Autodesk Fusion 360 part; units mm, degrees
(part 3 of 5)
  arc A39 (-57.6679, 11.8099) -> (-56.8988, 12.9306) centre (-57.8882, 12.7853) ccw
  arc A40 (-57.6679, 11.8099) -> (-58.5945, 11.5616) centre (-55, 0) ccw
  arc A41 (-59.8209, 12.1477) -> (-58.5945, 11.5616) centre (-58.8914, 12.5165) ccw
  line L20 (-59.8209, 12.1477) -> (-60.1994, 13.1014)
  spline S20 degree 5 poles (-60.1994, 13.1014) (-60.2031, 13.1108) (-60.2109, 13.1295) (-60.2234, 13.1571) (-60.2418, 13.1932) (-60.267, 13.2372) (-60.2939, 13.2804) (-60.3217, 13.3231) (-60.3501, 13.3657) (-60.3789, 13.408) (-60.4081, 13.4502) (-60.4379, 13.4921) (-60.4683, 13.5336) (-60.4995, 13.5747) (-60.5315, 13.6155) (-60.5642, 13.6558) (-60.5976, 13.6958) (-60.6314, 13.7355) (-60.6658, 13.775) (-60.7005, 13.8143) (-60.7357, 13.8532) (-60.7713, 13.8919) (-60.8074, 13.9304) (-60.844, 13.9685) (-60.8811, 14.0064) (-60.9187, 14.044) (-60.9566, 14.0813) (-60.995, 14.1184) (-61.0338, 14.1552) (-61.073, 14.1917) (-61.1126, 14.228) (-61.1525, 14.2641) (-61.1929, 14.2999) (-61.2336, 14.3354) (-61.2747, 14.3707) (-61.3161, 14.4057) (-61.358, 14.4405) (-61.4002, 14.4751) (-61.4427, 14.5093) (-61.4856, 14.5434) (-61.5288, 14.5772) (-61.5723, 14.6107) (-61.6162, 14.644) (-61.6604, 14.6771) (-61.7049, 14.7099) (-61.7498, 14.7424) (-61.7949, 14.7747) (-61.8404, 14.8068) (-61.8862, 14.8386) (-61.9323, 14.8702) (-61.9787, 14.9015) (-62.0253, 14.9326) (-62.0723, 14.9634) (-62.1196, 14.994) (-62.1672, 15.0244) (-62.215, 15.0545) (-62.2631, 15.0843) (-62.3115, 15.114) (-62.3602, 15.1433) (-62.4092, 15.1724) (-62.4584, 15.2013) (-62.5079, 15.2299) (-62.5577, 15.2583) (-62.6077, 15.2865) (-62.658, 15.3143) (-62.7085, 15.342) (-62.7594, 15.3694) (-62.8104, 15.3965) (-62.8617, 15.4234) (-62.9133, 15.4501) (-62.9651, 15.4765) (-63.0067, 15.4974) (-63.038, 15.513) (-63.059, 15.5233) (-63.0695, 15.5285) knots 0 0 0 0 0 0 0.01428571 0.02857143 0.04285714 0.05714286 0.07142857 0.08571429 0.1 0.11428571 0.12857143 0.14285714 0.15714286 0.17142857 0.18571429 0.2 0.21428571 0.22857143 0.24285714 0.25714286 0.27142857 0.28571429 0.3 0.31428571 0.32857143 0.34285714 0.35714286 0.37142857 0.38571429 0.4 0.41428571 0.42857143 0.44285714 0.45714286 0.47142857 0.48571429 0.5 0.51428571 0.52857143 0.54285714 0.55714286 0.57142857 0.58571429 0.6 0.61428571 0.62857143 0.64285714 0.65714286 0.67142857 0.68571429 0.7 0.71428571 0.72857143 0.74285714 0.75714286 0.77142857 0.78571429 0.8 0.81428571 0.82857143 0.84285714 0.85714286 0.87142857 0.88571429 0.9 0.91428571 0.92857143 0.94285714 0.95714286 0.97142857 0.98571429 1 1 1 1 1 1
  arc A42 (-63.0695, 15.5285) -> (-64.4133, 14.7526) centre (-55, 0) ccw
  spline S21 degree 5 poles (-64.4133, 14.7526) (-64.4141, 14.741) (-64.4156, 14.7176) (-64.4178, 14.6827) (-64.4205, 14.6362) (-64.4235, 14.5781) (-64.4262, 14.5202) (-64.4286, 14.4623) (-64.4306, 14.4045) (-64.4323, 14.3468) (-64.4336, 14.2892) (-64.4346, 14.2317) (-64.4353, 14.1743) (-64.4356, 14.117) (-64.4355, 14.0598) (-64.4351, 14.0028) (-64.4344, 13.9458) (-64.4333, 13.889) (-64.4319, 13.8322) (-64.4301, 13.7756) (-64.4279, 13.7191) (-64.4254, 13.6628) (-64.4226, 13.6065) (-64.4193, 13.5504) (-64.4158, 13.4945) (-64.4118, 13.4386) (-64.4075, 13.3829) (-64.4029, 13.3274) (-64.3978, 13.2719) (-64.3924, 13.2167) (-64.3867, 13.1616) (-64.3805, 13.1066) (-64.374, 13.0518) (-64.3671, 12.9971) (-64.3598, 12.9427) (-64.3522, 12.8883) (-64.3441, 12.8342) (-64.3357, 12.7802) (-64.3269, 12.7264) (-64.3177, 12.6728) (-64.3081, 12.6194) (-64.298, 12.5662) (-64.2876, 12.5131) (-64.2768, 12.4603) (-64.2655, 12.4077) (-64.2539, 12.3552) (-64.2418, 12.303) (-64.2293, 12.251) (-64.2164, 12.1993) (-64.2031, 12.1477) (-64.1893, 12.0964) (-64.1751, 12.0454) (-64.1603, 11.9946) (-64.1451, 11.9441) (-64.1294, 11.8939) (-64.1132, 11.8439) (-64.0966, 11.7942) (-64.0796, 11.7447) (-64.0621, 11.6955) (-64.0442, 11.6467) (-64.0256, 11.5981) (-64.0063, 11.5501) (-63.9863, 11.5025) (-63.9655, 11.4554) (-63.9441, 11.4087) (-63.9222, 11.3623) (-63.8999, 11.3162) (-63.8773, 11.2703) (-63.8542, 11.2248) (-63.8302, 11.1799) (-63.8047, 11.1361) (-63.7827, 11.1022) (-63.765, 11.0775) (-63.7527, 11.0614) (-63.7464, 11.0535) knots -1 -1 -1 -1 -1 -1 -0.98571429 -0.97142857 -0.95714286 -0.94285714 -0.92857143 -0.91428571 -0.9 -0.88571429 -0.87142857 -0.85714286 -0.84285714 -0.82857143 -0.81428571 -0.8 -0.78571429 -0.77142857 -0.75714286 -0.74285714 -0.72857143 -0.71428571 -0.7 -0.68571429 -0.67142857 -0.65714286 -0.64285714 -0.62857143 -0.61428571 -0.6 -0.58571429 -0.57142857 -0.55714286 -0.54285714 -0.52857143 -0.51428571 -0.5 -0.48571429 -0.47142857 -0.45714286 -0.44285714 -0.42857143 -0.41428571 -0.4 -0.38571429 -0.37142857 -0.35714286 -0.34285714 -0.32857143 -0.31428571 -0.3 -0.28571429 -0.27142857 -0.25714286 -0.24285714 -0.22857143 -0.21428571 -0.2 -0.18571429 -0.17142857 -0.15714286 -0.14285714 -0.12857143 -0.11428571 -0.1 -0.08571429 -0.07142857 -0.05714286 -0.04285714 -0.02857143 -0.01428571 0 0 0 0 0 0
  line L21 (-63.7464, 11.0535) -> (-63.1097, 10.2488)
  arc A43 (-63.2154, 8.8938) -> (-63.1097, 10.2488) centre (-63.8939, 9.6283) ccw
  arc A44 (-63.2154, 8.8938) -> (-63.8938, 8.2154) centre (-55, 0) ccw
  arc A45 (-65.2488, 8.1097) -> (-63.8938, 8.2154) centre (-64.6283, 8.8939) ccw
  line L22 (-65.2488, 8.1097) -> (-66.0535, 8.7464)
  spline S22 degree 5 poles (-66.0535, 8.7464) (-66.0614, 8.7527) (-66.0775, 8.765) (-66.1022, 8.7827) (-66.1361, 8.8047) (-66.1799, 8.8302) (-66.2248, 8.8542) (-66.2703, 8.8773) (-66.3162, 8.8999) (-66.3623, 8.9222) (-66.4087, 8.9441) (-66.4554, 8.9655) (-66.5025, 8.9863) (-66.5501, 9.0063) (-66.5981, 9.0256) (-66.6467, 9.0442) (-66.6955, 9.0621) (-66.7447, 9.0796) (-66.7942, 9.0966) (-66.8439, 9.1132) (-66.8939, 9.1294) (-66.9441, 9.1451) (-66.9946, 9.1603) (-67.0454, 9.1751) (-67.0964, 9.1893) (-67.1477, 9.2031) (-67.1993, 9.2164) (-67.251, 9.2293) (-67.303, 9.2418) (-67.3552, 9.2539) (-67.4077, 9.2655) (-67.4603, 9.2768) (-67.5131, 9.2876) (-67.5662, 9.298) (-67.6194, 9.3081) (-67.6728, 9.3177) (-67.7264, 9.3269) (-67.7802, 9.3357) (-67.8342, 9.3441) (-67.8883, 9.3522) (-67.9427, 9.3598) (-67.9971, 9.3671) (-68.0518, 9.374) (-68.1066, 9.3805) (-68.1616, 9.3867) (-68.2167, 9.3924) (-68.2719, 9.3978) (-68.3274, 9.4029) (-68.3829, 9.4075) (-68.4386, 9.4118) (-68.4945, 9.4158) (-68.5504, 9.4193) (-68.6065, 9.4226) (-68.6628, 9.4254) (-68.7191, 9.4279) (-68.7756, 9.4301) (-68.8322, 9.4319) (-68.889, 9.4333) (-68.9458, 9.4344) (-69.0028, 9.4351) (-69.0598, 9.4355) (-69.117, 9.4356) (-69.1743, 9.4353) (-69.2317, 9.4346) (-69.2892, 9.4336) (-69.3468, 9.4323) (-69.4045, 9.4306) (-69.4623, 9.4286) (-69.5202, 9.4262) (-69.5781, 9.4235) (-69.6362, 9.4205) (-69.6827, 9.4178) (-69.7176, 9.4156) (-69.741, 9.4141) (-69.7526, 9.4133) knots 0 0 0 0 0 0 0.01428571 0.02857143 0.04285714 0.05714286 0.07142857 0.08571429 0.1 0.11428571 0.12857143 0.14285714 0.15714286 0.17142857 0.18571429 0.2 0.21428571 0.22857143 0.24285714 0.25714286 0.27142857 0.28571429 0.3 0.31428571 0.32857143 0.34285714 0.35714286 0.37142857 0.38571429 0.4 0.41428571 0.42857143 0.44285714 0.45714286 0.47142857 0.48571429 0.5 0.51428571 0.52857143 0.54285714 0.55714286 0.57142857 0.58571429 0.6 0.61428571 0.62857143 0.64285714 0.65714286 0.67142857 0.68571429 0.7 0.71428571 0.72857143 0.74285714 0.75714286 0.77142857 0.78571429 0.8 0.81428571 0.82857143 0.84285714 0.85714286 0.87142857 0.88571429 0.9 0.91428571 0.92857143 0.94285714 0.95714286 0.97142857 0.98571429 1 1 1 1 1 1
  arc A46 (-69.7526, 9.4133) -> (-70.5285, 8.0695) centre (-55, 0) ccw
  spline S23 degree 5 poles (-70.5285, 8.0695) (-70.5233, 8.059) (-70.513, 8.038) (-70.4974, 8.0067) (-70.4765, 7.9651) (-70.4501, 7.9133) (-70.4234, 7.8617) (-70.3965, 7.8104) (-70.3694, 7.7594) (-70.342, 7.7085) (-70.3143, 7.658) (-70.2865, 7.6077) (-70.2583, 7.5577) (-70.2299, 7.5079) (-70.2013, 7.4584) (-70.1724, 7.4092) (-70.1433, 7.3602) (-70.114, 7.3115) (-70.0843, 7.2631) (-70.0545, 7.215) (-70.0244, 7.1672) (-69.994, 7.1196) (-69.9634, 7.0723) (-69.9326, 7.0253) (-69.9015, 6.9787) (-69.8702, 6.9323) (-69.8386, 6.8862) (-69.8068, 6.8404) (-69.7747, 6.7949) (-69.7424, 6.7498) (-69.7099, 6.7049) (-69.6771, 6.6604) (-69.644, 6.6162) (-69.6107, 6.5723) (-69.5772, 6.5288) (-69.5434, 6.4856) (-69.5093, 6.4427) (-69.4751, 6.4002) (-69.4405, 6.358) (-69.4057, 6.3161) (-69.3707, 6.2747) (-69.3354, 6.2336) (-69.2999, 6.1929) (-69.2641, 6.1525) (-69.228, 6.1126) (-69.1917, 6.073) (-69.1552, 6.0338) (-69.1184, 5.995) (-69.0813, 5.9566) (-69.044, 5.9187) (-69.0064, 5.8811) (-68.9685, 5.844) (-68.9304, 5.8074) (-68.8919, 5.7713) (-68.8532, 5.7357) (-68.8143, 5.7005) (-68.775, 5.6658) (-68.7355, 5.6314) (-68.6958, 5.5976) (-68.6558, 5.5642) (-68.6155, 5.5315) (-68.5747, 5.4995) (-68.5336, 5.4683) (-68.4921, 5.4379) (-68.4502, 5.4081) (-68.408, 5.3789) (-68.3657, 5.3501) (-68.3231, 5.3217) (-68.2804, 5.2939) (-68.2372, 5.267) (-68.1932, 5.2418) (-68.1571, 5.2234) (-68.1295, 5.2109) (-68.1108, 5.2031) (-68.1014, 5.1994) knots -1 -1 -1 -1 -1 -1 -0.98571429 -0.97142857 -0.95714286 -0.94285714 -0.92857143 -0.91428571 -0.9 -0.88571429 -0.87142857 -0.85714286 -0.84285714 -0.82857143 -0.81428571 -0.8 -0.78571429 -0.77142857 -0.75714286 -0.74285714 -0.72857143 -0.71428571 -0.7 -0.68571429 -0.67142857 -0.65714286 -0.64285714 -0.62857143 -0.61428571 -0.6 -0.58571429 -0.57142857 -0.55714286 -0.54285714 -0.52857143 -0.51428571 -0.5 -0.48571429 -0.47142857 -0.45714286 -0.44285714 -0.42857143 -0.41428571 -0.4 -0.38571429 -0.37142857 -0.35714286 -0.34285714 -0.32857143 -0.31428571 -0.3 -0.28571429 -0.27142857 -0.25714286 -0.24285714 -0.22857143 -0.21428571 -0.2 -0.18571429 -0.17142857 -0.15714286 -0.14285714 -0.12857143 -0.11428571 -0.1 -0.08571429 -0.07142857 -0.05714286 -0.04285714 -0.02857143 -0.01428571 0 0 0 0 0 0
  line L23 (-68.1014, 5.1994) -> (-67.1477, 4.8209)
  arc A47 (-66.5616, 3.5945) -> (-67.1477, 4.8209) centre (-67.5165, 3.8914) ccw
  circle A48 centre (-55, 0) radius 2.6
  line L24 (-50.5903, -1.85) -> (-59.4097, -1.85)
  line L25 (-59.4097, -1.85) -> (-59.4097, 1.85)
  line L26 (-59.4097, 1.85) -> (-50.5903, 1.85)
  line L27 (-50.5903, 1.85) -> (-50.5903, -1.85)
  line L28 (-50.5903, -1.85) -> (-59.4097, 1.85) construction
  line L29 (-59.4097, -1.85) -> (-50.5903, 1.85) construction
  circle A49 centre (-55, 0) radius 2.6
  point P0 (-55, 0)
  dimension "d49" = 3.7
  constraint horizontal L24
  constraint perpendicular L24 L25
  constraint parallel L24 L26
  constraint parallel L25 L27
  constraint coincident L28 P0
  constraint coincident L29 P0
  constraint coincident P0 A0.centre
  measures "d49" distance of L24.start L26.end
extrude "Extrude13" add sketch "Sketch20" against normal blind 3.3 contours A48 L24 A49 bodies 1
extrude "Extrude14" add sketch "Sketch20" against normal blind 3.3 contours A48 L26 A49 bodies 1
sketch "Sketch21" plane through (0, 0, 3.3) normal (0, 0, 1) x (-1, 0, 0)
  arc A0 (-136.8197, 3.9399) -> (-136.9255, 3.1358) centre (-110, 0) ccw
  arc A1 (-137.9991, 2.2547) -> (-136.9255, 3.1358) centre (-137.9188, 3.2515) ccw
  line L0 (-137.9991, 2.2547) -> (-138.0998, 2.2628)
  spline S0 degree 5 poles (-138.0998, 2.2628) (-138.1124, 2.2638) (-138.1377, 2.2655) (-138.1756, 2.2672) (-138.2262, 2.2675) (-138.2895, 2.2655) (-138.3528, 2.2616) (-138.4162, 2.2567) (-138.4797, 2.2511) (-138.5431, 2.2452) (-138.6066, 2.2388) (-138.67, 2.2319) (-138.7335, 2.2242) (-138.797, 2.2157) (-138.8605, 2.2063) (-138.9239, 2.1962) (-138.9874, 2.1853) (-139.0508, 2.1738) (-139.1143, 2.1619) (-139.1777, 2.1495) (-139.2411, 2.1366) (-139.3045, 2.1232) (-139.3679, 2.1093) (-139.4312, 2.0948) (-139.4946, 2.0798) (-139.5579, 2.0643) (-139.6212, 2.0484) (-139.6844, 2.0319) (-139.7477, 2.015) (-139.8109, 1.9977) (-139.8741, 1.98) (-139.9372, 1.9618) (-140.0003, 1.9432) (-140.0634, 1.9241) (-140.1264, 1.9047) (-140.1895, 1.8848) (-140.2524, 1.8645) (-140.3154, 1.8438) (-140.3783, 1.8227) (-140.4411, 1.8012) (-140.504, 1.7794) (-140.5667, 1.7571) (-140.6295, 1.7345) (-140.6922, 1.7115) (-140.7548, 1.6881) (-140.8174, 1.6644) (-140.88, 1.6402) (-140.9425, 1.6158) (-141.005, 1.5909) (-141.0674, 1.5658) (-141.1297, 1.5402) (-141.1921, 1.5143) (-141.2543, 1.4881) (-141.3165, 1.4615) (-141.3787, 1.4346) (-141.4408, 1.4073) (-141.5029, 1.3797) (-141.5649, 1.3518) (-141.6268, 1.3236) (-141.6887, 1.295) (-141.7505, 1.2661) (-141.8123, 1.2368) (-141.874, 1.2073) (-141.9356, 1.1774) (-141.9972, 1.1472) (-142.0588, 1.1167) (-142.1202, 1.0858) (-142.1816, 1.0547) (-142.243, 1.0233) (-142.3043, 0.9915) (-142.3655, 0.9594) (-142.4144, 0.9336) (-142.4511, 0.914) (-142.4755, 0.9009) (-142.4877, 0.8943) knots 0 0 0 0 0 0 0.01428571 0.02857143 0.04285714 0.05714286 0.07142857 0.08571429 0.1 0.11428571 0.12857143 0.14285714 0.15714286 0.17142857 0.18571429 0.2 0.21428571 0.22857143 0.24285714 0.25714286 0.27142857 0.28571429 0.3 0.31428571 0.32857143 0.34285714 0.35714286 0.37142857 0.38571429 0.4 0.41428571 0.42857143 0.44285714 0.45714286 0.47142857 0.48571429 0.5 0.51428571 0.52857143 0.54285714 0.55714286 0.57142857 0.58571429 0.6 0.61428571 0.62857143 0.64285714 0.65714286 0.67142857 0.68571429 0.7 0.71428571 0.72857143 0.74285714 0.75714286 0.77142857 0.78571429 0.8 0.81428571 0.82857143 0.84285714 0.85714286 0.87142857 0.88571429 0.9 0.91428571 0.92857143 0.94285714 0.95714286 0.97142857 0.98571429 1 1 1 1 1 1
  arc A2 (-142.4877, 0.8943) -> (-142.4877, -0.8943) centre (-110, 0) ccw
  spline S1 degree 5 poles (-142.4877, -0.8943) (-142.4755, -0.9009) (-142.4511, -0.914) (-142.4144, -0.9336) (-142.3655, -0.9594) (-142.3043, -0.9915) (-142.243, -1.0233) (-142.1816, -1.0547) (-142.1202, -1.0858) (-142.0588, -1.1167) (-141.9972, -1.1472) (-141.9356, -1.1774) (-141.874, -1.2073) (-141.8123, -1.2368) (-141.7505, -1.2661) (-141.6887, -1.295) (-141.6268, -1.3236) (-141.5649, -1.3518) (-141.5029, -1.3797) (-141.4408, -1.4073) (-141.3787, -1.4346) (-141.3165, -1.4615) (-141.2543, -1.4881) (-141.1921, -1.5143) (-141.1297, -1.5402) (-141.0674, -1.5658) (-141.005, -1.5909) (-140.9425, -1.6158) (-140.88, -1.6402) (-140.8174, -1.6644) (-140.7548, -1.6881) (-140.6922, -1.7115) (-140.6295, -1.7345) (-140.5667, -1.7571) (-140.504, -1.7794) (-140.4411, -1.8012) (-140.3783, -1.8227) (-140.3154, -1.8438) (-140.2524, -1.8645) (-140.1895, -1.8848) (-140.1264, -1.9047) (-140.0634, -1.9241) (-140.0003, -1.9432) (-139.9372, -1.9618) (-139.8741, -1.98) (-139.8109, -1.9977) (-139.7477, -2.015) (-139.6844, -2.0319) (-139.6212, -2.0484) (-139.5579, -2.0643) (-139.4946, -2.0798) (-139.4312, -2.0948) (-139.3679, -2.1093) (-139.3045, -2.1232) (-139.2411, -2.1366) (-139.1777, -2.1495) (-139.1143, -2.1619) (-139.0508, -2.1738) (-138.9874, -2.1853) (-138.9239, -2.1962) (-138.8605, -2.2063) (-138.797, -2.2157) (-138.7335, -2.2242) (-138.67, -2.2319) (-138.6066, -2.2388) (-138.5431, -2.2452) (-138.4797, -2.2511) (-138.4162, -2.2567) (-138.3528, -2.2616) (-138.2895, -2.2655) (-138.2262, -2.2675) (-138.1756, -2.2672) (-138.1377, -2.2655) (-138.1124, -2.2638) (-138.0998, -2.2628) knots -1 -1 -1 -1 -1 -1 -0.98571429 -0.97142857 -0.95714286 -0.94285714 -0.92857143 -0.91428571 -0.9 -0.88571429 -0.87142857 -0.85714286 -0.84285714 -0.82857143 -0.81428571 -0.8 -0.78571429 -0.77142857 -0.75714286 -0.74285714 -0.72857143 -0.71428571 -0.7 -0.68571429 -0.67142857 -0.65714286 -0.64285714 -0.62857143 -0.61428571 -0.6 -0.58571429 -0.57142857 -0.55714286 -0.54285714 -0.52857143 -0.51428571 -0.5 -0.48571429 -0.47142857 -0.45714286 -0.44285714 -0.42857143 -0.41428571 -0.4 -0.38571429 -0.37142857 -0.35714286 -0.34285714 -0.32857143 -0.31428571 -0.3 -0.28571429 -0.27142857 -0.25714286 -0.24285714 -0.22857143 -0.21428571 -0.2 -0.18571429 -0.17142857 -0.15714286 -0.14285714 -0.12857143 -0.11428571 -0.1 -0.08571429 -0.07142857 -0.05714286 -0.04285714 -0.02857143 -0.01428571 0 0 0 0 0 0
  line L1 (-138.0998, -2.2628) -> (-137.9991, -2.2547)
  arc A3 (-136.9255, -3.1358) -> (-137.9991, -2.2547) centre (-137.9188, -3.2515) ccw
  arc A4 (-136.9255, -3.1358) -> (-136.8197, -3.9399) centre (-110, 0) ccw
  arc A5 (-137.6286, -5.0688) -> (-136.8197, -3.9399) centre (-137.809, -4.0852) ccw
  line L2 (-137.6286, -5.0688) -> (-137.728, -5.0871)
  spline S2 degree 5 poles (-137.728, -5.0871) (-137.7405, -5.0893) (-137.7653, -5.0942) (-137.8023, -5.1025) (-137.8513, -5.1152) (-137.9119, -5.1336) (-137.9721, -5.1537) (-138.0321, -5.1749) (-138.0919, -5.1967) (-138.1516, -5.2188) (-138.2113, -5.2414) (-138.2708, -5.2645) (-138.3301, -5.2883) (-138.3892, -5.313) (-138.4481, -5.3385) (-138.5068, -5.3647) (-138.5653, -5.3917) (-138.6236, -5.4191) (-138.6818, -5.4471) (-138.7398, -5.4755) (-138.7977, -5.5044) (-138.8555, -5.5337) (-138.9131, -5.5636) (-138.9706, -5.5939) (-139.0279, -5.6248) (-139.085, -5.6561) (-139.142, -5.688) (-139.1989, -5.7202) (-139.2556, -5.7529) (-139.3121, -5.786) (-139.3686, -5.8195) (-139.4249, -5.8534) (-139.481, -5.8877) (-139.537, -5.9224) (-139.5929, -5.9575) (-139.6486, -5.9931) (-139.7042, -6.029) (-139.7596, -6.0652) (-139.8149, -6.1019) (-139.8701, -6.1389) (-139.9251, -6.1763) (-139.98, -6.214) (-140.0347, -6.2521) (-140.0893, -6.2906) (-140.1438, -6.3293) (-140.1981, -6.3685) (-140.2523, -6.408) (-140.3063, -6.4478) (-140.3603, -6.4879) (-140.414, -6.5284) (-140.4677, -6.5692) (-140.5212, -6.6104) (-140.5745, -6.6518) (-140.6277, -6.6936) (-140.6808, -6.7357) (-140.7337, -6.7781) (-140.7865, -6.8208) (-140.8392, -6.8638) (-140.8917, -6.9072) (-140.9441, -6.9508) (-140.9963, -6.9947) (-141.0484, -7.0389) (-141.1004, -7.0835) (-141.1522, -7.1283) (-141.2039, -7.1734) (-141.2554, -7.2188) (-141.3068, -7.2645) (-141.3581, -7.3104) (-141.4092, -7.3567) (-141.4601, -7.4032) (-141.511, -7.45) (-141.5515, -7.4877) (-141.5819, -7.5161) (-141.6021, -7.5351) (-141.6122, -7.5446) knots 0 0 0 0 0 0 0.01428571 0.02857143 0.04285714 0.05714286 0.07142857 0.08571429 0.1 0.11428571 0.12857143 0.14285714 0.15714286 0.17142857 0.18571429 0.2 0.21428571 0.22857143 0.24285714 0.25714286 0.27142857 0.28571429 0.3 0.31428571 0.32857143 0.34285714 0.35714286 0.37142857 0.38571429 0.4 0.41428571 0.42857143 0.44285714 0.45714286 0.47142857 0.48571429 0.5 0.51428571 0.52857143 0.54285714 0.55714286 0.57142857 0.58571429 0.6 0.61428571 0.62857143 0.64285714 0.65714286 0.67142857 0.68571429 0.7 0.71428571 0.72857143 0.74285714 0.75714286 0.77142857 0.78571429 0.8 0.81428571 0.82857143 0.84285714 0.85714286 0.87142857 0.88571429 0.9 0.91428571 0.92857143 0.94285714 0.95714286 0.97142857 0.98571429 1 1 1 1 1 1
  arc A6 (-141.6122, -7.5446) -> (-141.1492, -9.2723) centre (-110, 0) ccw
  spline S3 degree 5 poles (-141.1492, -9.2723) (-141.1357, -9.2755) (-141.1088, -9.2818) (-141.0683, -9.2912) (-141.0143, -9.3036) (-140.9469, -9.3187) (-140.8795, -9.3335) (-140.8121, -9.348) (-140.7447, -9.3622) (-140.6774, -9.376) (-140.61, -9.3896) (-140.5427, -9.4028) (-140.4755, -9.4157) (-140.4082, -9.4283) (-140.341, -9.4406) (-140.2738, -9.4525) (-140.2066, -9.4641) (-140.1394, -9.4753) (-140.0723, -9.4863) (-140.0052, -9.4969) (-139.9382, -9.5071) (-139.8712, -9.517) (-139.8042, -9.5266) (-139.7373, -9.5358) (-139.6704, -9.5447) (-139.6035, -9.5532) (-139.5367, -9.5614) (-139.47, -9.5692) (-139.4032, -9.5767) (-139.3366, -9.5838) (-139.27, -9.5905) (-139.2034, -9.5969) (-139.1369, -9.6029) (-139.0704, -9.6085) (-139.004, -9.6137) (-138.9377, -9.6186) (-138.8714, -9.6231) (-138.8052, -9.6272) (-138.739, -9.6309) (-138.673, -9.6342) (-138.607, -9.6371) (-138.541, -9.6395) (-138.4752, -9.6416) (-138.4094, -9.6432) (-138.3437, -9.6445) (-138.2781, -9.6453) (-138.2125, -9.6456) (-138.1471, -9.6456) (-138.0817, -9.6451) (-138.0164, -9.6441) (-137.9513, -9.6427) (-137.8862, -9.6408) (-137.8213, -9.6384) (-137.7565, -9.6354) (-137.6918, -9.6319) (-137.6272, -9.628) (-137.5627, -9.6235) (-137.4983, -9.6187) (-137.4341, -9.6133) (-137.37, -9.6074) (-137.306, -9.6008) (-137.2423, -9.5934) (-137.1788, -9.5852) (-137.1155, -9.5762) (-137.0524, -9.5665) (-136.9894, -9.5562) (-136.9266, -9.5455) (-136.8639, -9.5344) (-136.8014, -9.5228) (-136.7392, -9.5101) (-136.6775, -9.4957) (-136.6288, -9.4823) (-136.5926, -9.4709) (-136.5686, -9.4627) (-136.5567, -9.4585) knots -1 -1 -1 -1 -1 -1 -0.98571429 -0.97142857 -0.95714286 -0.94285714 -0.92857143 -0.91428571 -0.9 -0.88571429 -0.87142857 -0.85714286 -0.84285714 -0.82857143 -0.81428571 -0.8 -0.78571429 -0.77142857 -0.75714286 -0.74285714 -0.72857143 -0.71428571 -0.7 -0.68571429 -0.67142857 -0.65714286 -0.64285714 -0.62857143 -0.61428571 -0.6 -0.58571429 -0.57142857 -0.55714286 -0.54285714 -0.52857143 -0.51428571 -0.5 -0.48571429 -0.47142857 -0.45714286 -0.44285714 -0.42857143 -0.41428571 -0.4 -0.38571429 -0.37142857 -0.35714286 -0.34285714 -0.32857143 -0.31428571 -0.3 -0.28571429 -0.27142857 -0.25714286 -0.24285714 -0.22857143 -0.21428571 -0.2 -0.18571429 -0.17142857 -0.15714286 -0.14285714 -0.12857143 -0.11428571 -0.1 -0.08571429 -0.07142857 -0.05714286 -0.04285714 -0.02857143 -0.01428571 0 0 0 0 0 0
  line L3 (-136.5567, -9.4585) -> (-136.4615, -9.4246)
  arc A7 (-135.1964, -9.9978) -> (-136.4615, -9.4246) centre (-136.1259, -10.3666) ccw
  arc A8 (-135.1964, -9.9978) -> (-134.8861, -10.7471) centre (-110, 0) ccw
  arc A9 (-135.3753, -12.0469) -> (-134.8861, -10.7471) centre (-135.8041, -11.1435) ccw
  line L4 (-135.3753, -12.0469) -> (-135.4666, -12.0903)
  spline S4 degree 5 poles (-135.4666, -12.0903) (-135.478, -12.0957) (-135.5007, -12.1068) (-135.5344, -12.1244) (-135.5783, -12.1494) (-135.6321, -12.1828) (-135.6851, -12.2178) (-135.7375, -12.2538) (-135.7897, -12.2903) (-135.8417, -12.3272) (-135.8934, -12.3644) (-135.9449, -12.4021) (-135.9961, -12.4405) (-136.0468, -12.4796) (-136.0971, -12.5195) (-136.1469, -12.56) (-136.1965, -12.6012) (-136.2457, -12.6428) (-136.2946, -12.6849) (-136.3434, -12.7274) (-136.3918, -12.7702) (-136.44, -12.8135) (-136.488, -12.8573) (-136.5356, -12.9015) (-136.583, -12.9461) (-136.6301, -12.9912) (-136.6769, -13.0367) (-136.7234, -13.0825) (-136.7698, -13.1288) (-136.8158, -13.1754) (-136.8617, -13.2223) (-136.9073, -13.2697) (-136.9526, -13.3173) (-136.9977, -13.3654) (-137.0426, -13.4137) (-137.0872, -13.4625) (-137.1316, -13.5115) (-137.1758, -13.5609) (-137.2197, -13.6106) (-137.2634, -13.6607) (-137.3069, -13.711) (-137.3501, -13.7617) (-137.3931, -13.8126) (-137.4359, -13.8639) (-137.4785, -13.9155) (-137.5208, -13.9673) (-137.563, -14.0195) (-137.6049, -14.0719) (-137.6466, -14.1247) (-137.688, -14.1777) (-137.7293, -14.231) (-137.7703, -14.2846) (-137.8111, -14.3384) (-137.8517, -14.3926) (-137.892, -14.4469) (-137.9322, -14.5016) (-137.9721, -14.5565) (-138.0119, -14.6117) (-138.0514, -14.6672) (-138.0907, -14.7229) (-138.1298, -14.7788) (-138.1687, -14.835) (-138.2073, -14.8915) (-138.2458, -14.9482) (-138.284, -15.0051) (-138.322, -15.0623) (-138.3599, -15.1197) (-138.3975, -15.1774) (-138.4349, -15.2353) (-138.4721, -15.2935) (-138.509, -15.3518) (-138.5385, -15.3987) (-138.5604, -15.434) (-138.575, -15.4575) (-138.5823, -15.4693) knots 0 0 0 0 0 0 0.01428571 0.02857143 0.04285714 0.05714286 0.07142857 0.08571429 0.1 0.11428571 0.12857143 0.14285714 0.15714286 0.17142857 0.18571429 0.2 0.21428571 0.22857143 0.24285714 0.25714286 0.27142857 0.28571429 0.3 0.31428571 0.32857143 0.34285714 0.35714286 0.37142857 0.38571429 0.4 0.41428571 0.42857143 0.44285714 0.45714286 0.47142857 0.48571429 0.5 0.51428571 0.52857143 0.54285714 0.55714286 0.57142857 0.58571429 0.6 0.61428571 0.62857143 0.64285714 0.65714286 0.67142857 0.68571429 0.7 0.71428571 0.72857143 0.74285714 0.75714286 0.77142857 0.78571429 0.8 0.81428571 0.82857143 0.84285714 0.85714286 0.87142857 0.88571429 0.9 0.91428571 0.92857143 0.94285714 0.95714286 0.97142857 0.98571429 1 1 1 1 1 1
  arc A10 (-138.5823, -15.4693) -> (-137.688, -17.0184) centre (-110, 0) ccw
  spline S5 degree 5 poles (-137.688, -17.0184) (-137.6741, -17.0179) (-137.6464, -17.0171) (-137.6049, -17.0157) (-137.5496, -17.0136) (-137.4806, -17.0108) (-137.4116, -17.0077) (-137.3428, -17.0042) (-137.274, -17.0005) (-137.2054, -16.9965) (-137.1368, -16.9921) (-137.0684, -16.9875) (-137.0001, -16.9825) (-136.9318, -16.9773) (-136.8637, -16.9717) (-136.7957, -16.9658) (-136.7278, -16.9596) (-136.6601, -16.9531) (-136.5924, -16.9463) (-136.5249, -16.9392) (-136.4574, -16.9317) (-136.3902, -16.924) (-136.323, -16.9159) (-136.2559, -16.9075) (-136.189, -16.8987) (-136.1223, -16.8897) (-136.0556, -16.8803) (-135.9891, -16.8705) (-135.9227, -16.8605) (-135.8565, -16.8501) (-135.7904, -16.8393) (-135.7245, -16.8283) (-135.6587, -16.8168) (-135.593, -16.8051) (-135.5275, -16.7929) (-135.4622, -16.7805) (-135.397, -16.7676) (-135.332, -16.7545) (-135.2671, -16.7409) (-135.2025, -16.727) (-135.1379, -16.7127) (-135.0736, -16.698) (-135.0095, -16.683) (-134.9455, -16.6676) (-134.8817, -16.6517) (-134.8181, -16.6355) (-134.7547, -16.6189) (-134.6915, -16.6019) (-134.6285, -16.5845) (-134.5657, -16.5667) (-134.5031, -16.5485) (-134.4408, -16.5298) (-134.3787, -16.5106) (-134.3169, -16.491) (-134.2553, -16.4709) (-134.1939, -16.4503) (-134.1328, -16.4294) (-134.0718, -16.408) (-134.0112, -16.3862) (-133.9508, -16.3639) (-133.8907, -16.341) (-133.8311, -16.3174) (-133.7718, -16.293) (-133.713, -16.2679) (-133.6546, -16.2422) (-133.5965, -16.2159) (-133.5386, -16.1894) (-133.4809, -16.1625) (-133.4235, -16.135) (-133.3667, -16.1067) (-133.3108, -16.0768) (-133.2672, -16.0512) (-133.2352, -16.0309) (-133.2142, -16.0168) (-133.2037, -16.0096) knots -1 -1 -1 -1 -1 -1 -0.98571429 -0.97142857 -0.95714286 -0.94285714 -0.92857143 -0.91428571 -0.9 -0.88571429 -0.87142857 -0.85714286 -0.84285714 -0.82857143 -0.81428571 -0.8 -0.78571429 -0.77142857 -0.75714286 -0.74285714 -0.72857143 -0.71428571 -0.7 -0.68571429 -0.67142857 -0.65714286 -0.64285714 -0.62857143 -0.61428571 -0.6 -0.58571429 -0.57142857 -0.55714286 -0.54285714 -0.52857143 -0.51428571 -0.5 -0.48571429 -0.47142857 -0.45714286 -0.44285714 -0.42857143 -0.41428571 -0.4 -0.38571429 -0.37142857 -0.35714286 -0.34285714 -0.32857143 -0.31428571 -0.3 -0.28571429 -0.27142857 -0.25714286 -0.24285714 -0.22857143 -0.21428571 -0.2 -0.18571429 -0.17142857 -0.15714286 -0.14285714 -0.12857143 -0.11428571 -0.1 -0.08571429 -0.07142857 -0.05714286 -0.04285714 -0.02857143 -0.01428571 0 0 0 0 0 0
  line L5 (-133.2037, -16.0096) -> (-133.1206, -15.9522)
  arc A11 (-131.7503, -16.1784) -> (-133.1206, -15.9522) centre (-132.5527, -16.7753) ccw
  arc A12 (-131.7503, -16.1784) -> (-131.2566, -16.8219) centre (-110, 0) ccw
  arc A13 (-131.3926, -18.204) -> (-131.2566, -16.8219) centre (-132.0407, -17.4424) ccw
  line L6 (-131.3926, -18.204) -> (-131.4696, -18.2695)
  spline S6 degree 5 poles (-131.4696, -18.2695) (-131.4793, -18.2777) (-131.4983, -18.2944) (-131.5263, -18.32) (-131.5623, -18.3556) (-131.6056, -18.4018) (-131.6477, -18.4493) (-131.689, -18.4976) (-131.73, -18.5464) (-131.7706, -18.5954) (-131.811, -18.6448) (-131.851, -18.6946) (-131.8904, -18.7449) (-131.9293, -18.7958) (-131.9675, -18.8473) (-132.0052, -18.8994) (-132.0424, -18.9519) (-132.0792, -19.0049) (-132.1156, -19.0582) (-132.1516, -19.1119) (-132.1874, -19.1658) (-132.2227, -19.2201) (-132.2577, -19.2748) (-132.2923, -19.3298) (-132.3265, -19.3852) (-132.3603, -19.4409) (-132.3937, -19.4969) (-132.4268, -19.5533) (-132.4596, -19.6099) (-132.4921, -19.6669) (-132.5242, -19.7241) (-132.556, -19.7816) (-132.5875, -19.8394) (-132.6186, -19.8975) (-132.6494, -19.9558) (-132.6799, -20.0144) (-132.7101, -20.0733) (-132.74, -20.1325) (-132.7695, -20.1918) (-132.7988, -20.2515) (-132.8277, -20.3114) (-132.8564, -20.3715) (-132.8848, -20.4318) (-132.9128, -20.4924) (-132.9406, -20.5533) (-132.9681, -20.6143) (-132.9953, -20.6756) (-133.0222, -20.7371) (-133.0488, -20.7988) (-133.0751, -20.8608) (-133.1011, -20.923) (-133.1269, -20.9853) (-133.1524, -21.0479) (-133.1776, -21.1107) (-133.2025, -21.1737) (-133.2271, -21.2369) (-133.2515, -21.3003) (-133.2756, -21.3638) (-133.2994, -21.4276) (-133.323, -21.4916) (-133.3462, -21.5558) (-133.3693, -21.6201) (-133.392, -21.6847) (-133.4145, -21.7494) (-133.4367, -21.8143) (-133.4586, -21.8794) (-133.4803, -21.9446) (-133.5017, -22.0101) (-133.5228, -22.0757) (-133.5437, -22.1415) (-133.5643, -22.2074) (-133.5806, -22.2603) (-133.5927, -22.3001) (-133.6007, -22.3266) (-133.6047, -22.3399) knots 0 0 0 0 0 0 0.01428571 0.02857143 0.04285714 0.05714286 0.07142857 0.08571429 0.1 0.11428571 0.12857143 0.14285714 0.15714286 0.17142857 0.18571429 0.2 0.21428571 0.22857143 0.24285714 0.25714286 0.27142857 0.28571429 0.3 0.31428571 0.32857143 0.34285714 0.35714286 0.37142857 0.38571429 0.4 0.41428571 0.42857143 0.44285714 0.45714286 0.47142857 0.48571429 0.5 0.51428571 0.52857143 0.54285714 0.55714286 0.57142857 0.58571429 0.6 0.61428571 0.62857143 0.64285714 0.65714286 0.67142857 0.68571429 0.7 0.71428571 0.72857143 0.74285714 0.75714286 0.77142857 0.78571429 0.8 0.81428571 0.82857143 0.84285714 0.85714286 0.87142857 0.88571429 0.9 0.91428571 0.92857143 0.94285714 0.95714286 0.97142857 0.98571429 1 1 1 1 1 1
  arc A14 (-133.6047, -22.3399) -> (-132.3399, -23.6047) centre (-110, 0) ccw
  spline S7 degree 5 poles (-132.3399, -23.6047) (-132.3266, -23.6007) (-132.3001, -23.5927) (-132.2603, -23.5806) (-132.2074, -23.5643) (-132.1415, -23.5437) (-132.0757, -23.5228) (-132.0101, -23.5017) (-131.9446, -23.4803) (-131.8794, -23.4586) (-131.8143, -23.4367) (-131.7494, -23.4145) (-131.6847, -23.392) (-131.6201, -23.3693) (-131.5558, -23.3462) (-131.4916, -23.323) (-131.4276, -23.2994) (-131.3638, -23.2756) (-131.3003, -23.2515) (-131.2369, -23.2271) (-131.1737, -23.2025) (-131.1107, -23.1776) (-131.0479, -23.1524) (-130.9853, -23.1269) (-130.923, -23.1011) (-130.8608, -23.0751) (-130.7988, -23.0488) (-130.7371, -23.0222) (-130.6756, -22.9953) (-130.6143, -22.9681) (-130.5533, -22.9406) (-130.4924, -22.9128) (-130.4318, -22.8848) (-130.3715, -22.8564) (-130.3114, -22.8277) (-130.2515, -22.7988) (-130.1918, -22.7695) (-130.1325, -22.74) (-130.0733, -22.7101) (-130.0144, -22.6799) (-129.9558, -22.6494) (-129.8975, -22.6186) (-129.8394, -22.5875) (-129.7816, -22.556) (-129.7241, -22.5242) (-129.6669, -22.4921) (-129.6099, -22.4596) (-129.5533, -22.4268) (-129.4969, -22.3937) (-129.4409, -22.3603) (-129.3852, -22.3265) (-129.3298, -22.2923) (-129.2748, -22.2577) (-129.2201, -22.2227) (-129.1658, -22.1874) (-129.1119, -22.1516) (-129.0582, -22.1156) (-129.0049, -22.0792) (-128.9519, -22.0424) (-128.8994, -22.0052) (-128.8473, -21.9675) (-128.7958, -21.9293) (-128.7449, -21.8904) (-128.6946, -21.851) (-128.6448, -21.811) (-128.5954, -21.7706) (-128.5464, -21.73) (-128.4976, -21.689) (-128.4493, -21.6477) (-128.4018, -21.6056) (-128.3556, -21.5623) (-128.32, -21.5263) (-128.2944, -21.4983) (-128.2777, -21.4793) (-128.2695, -21.4696) knots -1 -1 -1 -1 -1 -1 -0.98571429 -0.97142857 -0.95714286 -0.94285714 -0.92857143 -0.91428571 -0.9 -0.88571429 -0.87142857 -0.85714286 -0.84285714 -0.82857143 -0.81428571 -0.8 -0.78571429 -0.77142857 -0.75714286 -0.74285714 -0.72857143 -0.71428571 -0.7 -0.68571429 -0.67142857 -0.65714286 -0.64285714 -0.62857143 -0.61428571 -0.6 -0.58571429 -0.57142857 -0.55714286 -0.54285714 -0.52857143 -0.51428571 -0.5 -0.48571429 -0.47142857 -0.45714286 -0.44285714 -0.42857143 -0.41428571 -0.4 -0.38571429 -0.37142857 -0.35714286 -0.34285714 -0.32857143 -0.31428571 -0.3 -0.28571429 -0.27142857 -0.25714286 -0.24285714 -0.22857143 -0.21428571 -0.2 -0.18571429 -0.17142857 -0.15714286 -0.14285714 -0.12857143 -0.11428571 -0.1 -0.08571429 -0.07142857 -0.05714286 -0.04285714 -0.02857143 -0.01428571 0 0 0 0 0 0
  line L7 (-128.2695, -21.4696) -> (-128.204, -21.3926)
  arc A15 (-126.8219, -21.2566) -> (-128.204, -21.3926) centre (-127.4424, -22.0407) ccw
  arc A16 (-126.8219, -21.2566) -> (-126.1784, -21.7503) centre (-110, 0) ccw
  arc A17 (-125.9522, -23.1206) -> (-126.1784, -21.7503) centre (-126.7753, -22.5527) ccw
  line L8 (-125.9522, -23.1206) -> (-126.0096, -23.2037)
  spline S8 degree 5 poles (-126.0096, -23.2037) (-126.0168, -23.2142) (-126.0309, -23.2352) (-126.0512, -23.2672) (-126.0768, -23.3108) (-126.1067, -23.3667) (-126.135, -23.4235) (-126.1625, -23.4809) (-126.1894, -23.5386) (-126.2159, -23.5965) (-126.2422, -23.6546) (-126.2679, -23.713) (-126.293, -23.7718) (-126.3174, -23.8311) (-126.341, -23.8907) (-126.3639, -23.9508) (-126.3862, -24.0112) (-126.408, -24.0718) (-126.4294, -24.1328) (-126.4503, -24.1939) (-126.4709, -24.2553) (-126.491, -24.3169) (-126.5106, -24.3787) (-126.5298, -24.4408) (-126.5485, -24.5031) (-126.5667, -24.5657) (-126.5845, -24.6285) (-126.6019, -24.6915) (-126.6189, -24.7547) (-126.6355, -24.8181) (-126.6517, -24.8817) (-126.6676, -24.9455) (-126.683, -25.0095) (-126.698, -25.0736) (-126.7127, -25.1379) (-126.727, -25.2025) (-126.7409, -25.2671) (-126.7545, -25.332) (-126.7676, -25.397) (-126.7805, -25.4622) (-126.7929, -25.5275) (-126.8051, -25.593) (-126.8168, -25.6587) (-126.8283, -25.7245) (-126.8393, -25.7904) (-126.8501, -25.8565) (-126.8605, -25.9227) (-126.8705, -25.9891) (-126.8803, -26.0556) (-126.8897, -26.1223) (-126.8987, -26.189) (-126.9075, -26.2559) (-126.9159, -26.323) (-126.924, -26.3902) (-126.9317, -26.4574) (-126.9392, -26.5249) (-126.9463, -26.5924) (-126.9531, -26.6601) (-126.9596, -26.7278) (-126.9658, -26.7957) (-126.9717, -26.8637) (-126.9773, -26.9318) (-126.9825, -27.0001) (-126.9875, -27.0684) (-126.9921, -27.1368) (-126.9965, -27.2054) (-127.0005, -27.274) (-127.0042, -27.3428) (-127.0077, -27.4116) (-127.0108, -27.4806) (-127.0136, -27.5496) (-127.0157, -27.6049) (-127.0171, -27.6464) (-127.0179, -27.6741) (-127.0184, -27.688) knots 0 0 0 0 0 0 0.01428571 0.02857143 0.04285714 0.05714286 0.07142857 0.08571429 0.1 0.11428571 0.12857143 0.14285714 0.15714286 0.17142857 0.18571429 0.2 0.21428571 0.22857143 0.24285714 0.25714286 0.27142857 0.28571429 0.3 0.31428571 0.32857143 0.34285714 0.35714286 0.37142857 0.38571429 0.4 0.41428571 0.42857143 0.44285714 0.45714286 0.47142857 0.48571429 0.5 0.51428571 0.52857143 0.54285714 0.55714286 0.57142857 0.58571429 0.6 0.61428571 0.62857143 0.64285714 0.65714286 0.67142857 0.68571429 0.7 0.71428571 0.72857143 0.74285714 0.75714286 0.77142857 0.78571429 0.8 0.81428571 0.82857143 0.84285714 0.85714286 0.87142857 0.88571429 0.9 0.91428571 0.92857143 0.94285714 0.95714286 0.97142857 0.98571429 1 1 1 1 1 1
  arc A18 (-127.0184, -27.688) -> (-125.4693, -28.5823) centre (-110, 0) ccw
  spline S9 degree 5 poles (-125.4693, -28.5823) (-125.4575, -28.575) (-125.434, -28.5604) (-125.3987, -28.5385) (-125.3518, -28.509) (-125.2935, -28.4721) (-125.2353, -28.4349) (-125.1774, -28.3975) (-125.1197, -28.3599) (-125.0623, -28.322) (-125.0051, -28.284) (-124.9482, -28.2458) (-124.8915, -28.2073) (-124.835, -28.1687) (-124.7788, -28.1298) (-124.7229, -28.0907) (-124.6672, -28.0514) (-124.6117, -28.0119) (-124.5565, -27.9721) (-124.5016, -27.9322) (-124.4469, -27.892) (-124.3926, -27.8517) (-124.3384, -27.8111) (-124.2846, -27.7703) (-124.231, -27.7293) (-124.1777, -27.688) (-124.1247, -27.6466) (-124.0719, -27.6049) (-124.0195, -27.563) (-123.9673, -27.5208) (-123.9155, -27.4785) (-123.8639, -27.4359) (-123.8126, -27.3931) (-123.7617, -27.3501) (-123.711, -27.3069) (-123.6607, -27.2634) (-123.6106, -27.2197) (-123.5609, -27.1758) (-123.5115, -27.1316) (-123.4625, -27.0872) (-123.4137, -27.0426) (-123.3654, -26.9977) (-123.3173, -26.9526) (-123.2697, -26.9073) (-123.2223, -26.8617) (-123.1754, -26.8158) (-123.1288, -26.7698) (-123.0825, -26.7234) (-123.0367, -26.6769) (-122.9912, -26.6301) (-122.9461, -26.583) (-122.9015, -26.5356) (-122.8573, -26.488) (-122.8135, -26.44) (-122.7702, -26.3918) (-122.7274, -26.3434) (-122.6849, -26.2946) (-122.6428, -26.2457) (-122.6012, -26.1965) (-122.56, -26.1469) (-122.5195, -26.0971) (-122.4796, -26.0468) (-122.4405, -25.9961) (-122.4021, -25.9449) (-122.3644, -25.8934) (-122.3272, -25.8417) (-122.2903, -25.7897) (-122.2538, -25.7375) (-122.2178, -25.6851) (-122.1828, -25.6321) (-122.1494, -25.5783) (-122.1244, -25.5344) (-122.1068, -25.5007) (-122.0957, -25.478) (-122.0903, -25.4666) knots -1 -1 -1 -1 -1 -1 -0.98571429 -0.97142857 -0.95714286 -0.94285714 -0.92857143 -0.91428571 -0.9 -0.88571429 -0.87142857 -0.85714286 -0.84285714 -0.82857143 -0.81428571 -0.8 -0.78571429 -0.77142857 -0.75714286 -0.74285714 -0.72857143 -0.71428571 -0.7 -0.68571429 -0.67142857 -0.65714286 -0.64285714 -0.62857143 -0.61428571 -0.6 -0.58571429 -0.57142857 -0.55714286 -0.54285714 -0.52857143 -0.51428571 -0.5 -0.48571429 -0.47142857 -0.45714286 -0.44285714 -0.42857143 -0.41428571 -0.4 -0.38571429 -0.37142857 -0.35714286 -0.34285714 -0.32857143 -0.31428571 -0.3 -0.28571429 -0.27142857 -0.25714286 -0.24285714 -0.22857143 -0.21428571 -0.2 -0.18571429 -0.17142857 -0.15714286 -0.14285714 -0.12857143 -0.11428571 -0.1 -0.08571429 -0.07142857 -0.05714286 -0.04285714 -0.02857143 -0.01428571 0 0 0 0 0 0
  line L9 (-122.0903, -25.4666) -> (-122.0469, -25.3753)
  arc A19 (-120.7471, -24.8861) -> (-122.0469, -25.3753) centre (-121.1435, -25.8041) ccw
  arc A20 (-120.7471, -24.8861) -> (-119.9978, -25.1964) centre (-110, 0) ccw
  arc A21 (-119.4246, -26.4615) -> (-119.9978, -25.1964) centre (-120.3666, -26.1259) ccw
  line L10 (-119.4246, -26.4615) -> (-119.4585, -26.5567)
  spline S10 degree 5 poles (-119.4585, -26.5567) (-119.4627, -26.5686) (-119.4709, -26.5926) (-119.4823, -26.6288) (-119.4957, -26.6775) (-119.5101, -26.7392) (-119.5228, -26.8014) (-119.5344, -26.8639) (-119.5455, -26.9266) (-119.5562, -26.9894) (-119.5665, -27.0524) (-119.5762, -27.1155) (-119.5852, -27.1788) (-119.5934, -27.2423) (-119.6008, -27.306) (-119.6074, -27.37) (-119.6133, -27.4341) (-119.6187, -27.4983) (-119.6235, -27.5627) (-119.628, -27.6272) (-119.6319, -27.6918) (-119.6354, -27.7565) (-119.6384, -27.8213) (-119.6408, -27.8862) (-119.6427, -27.9513) (-119.6441, -28.0164) (-119.6451, -28.0817) (-119.6456, -28.1471) (-119.6456, -28.2125) (-119.6453, -28.2781) (-119.6445, -28.3437) (-119.6432, -28.4094) (-119.6416, -28.4752) (-119.6395, -28.541) (-119.6371, -28.607) (-119.6342, -28.673) (-119.6309, -28.739) (-119.6272, -28.8052) (-119.6231, -28.8714) (-119.6186, -28.9377) (-119.6137, -29.004) (-119.6085, -29.0704) (-119.6029, -29.1369) (-119.5969, -29.2034) (-119.5905, -29.27) (-119.5838, -29.3366) (-119.5767, -29.4032) (-119.5692, -29.47) (-119.5614, -29.5367) (-119.5532, -29.6035) (-119.5447, -29.6704) (-119.5358, -29.7373) (-119.5266, -29.8042) (-119.517, -29.8712) (-119.5071, -29.9382) (-119.4969, -30.0052) (-119.4863, -30.0723) (-119.4753, -30.1394) (-119.4641, -30.2066) (-119.4525, -30.2738) (-119.4406, -30.341) (-119.4283, -30.4082) (-119.4157, -30.4755) (-119.4028, -30.5427) (-119.3896, -30.61) (-119.376, -30.6774) (-119.3622, -30.7447) (-119.348, -30.8121) (-119.3335, -30.8795) (-119.3187, -30.9469) (-119.3036, -31.0143) (-119.2912, -31.0683) (-119.2818, -31.1088) (-119.2755, -31.1357) (-119.2723, -31.1492) knots 0 0 0 0 0 0 0.01428571 0.02857143 0.04285714 0.05714286 0.07142857 0.08571429 0.1 0.11428571 0.12857143 0.14285714 0.15714286 0.17142857 0.18571429 0.2 0.21428571 0.22857143 0.24285714 0.25714286 0.27142857 0.28571429 0.3 0.31428571 0.32857143 0.34285714 0.35714286 0.37142857 0.38571429 0.4 0.41428571 0.42857143 0.44285714 0.45714286 0.47142857 0.48571429 0.5 0.51428571 0.52857143 0.54285714 0.55714286 0.57142857 0.58571429 0.6 0.61428571 0.62857143 0.64285714 0.65714286 0.67142857 0.68571429 0.7 0.71428571 0.72857143 0.74285714 0.75714286 0.77142857 0.78571429 0.8 0.81428571 0.82857143 0.84285714 0.85714286 0.87142857 0.88571429 0.9 0.91428571 0.92857143 0.94285714 0.95714286 0.97142857 0.98571429 1 1 1 1 1 1
  arc A22 (-119.2723, -31.1492) -> (-117.5446, -31.6122) centre (-110, 0) ccw
  spline S11 degree 5 poles (-117.5446, -31.6122) (-117.5351, -31.6021) (-117.5161, -31.5819) (-117.4877, -31.5515) (-117.45, -31.511) (-117.4032, -31.4601) (-117.3567, -31.4092) (-117.3104, -31.3581) (-117.2645, -31.3068) (-117.2188, -31.2554) (-117.1734, -31.2039) (-117.1283, -31.1522) (-117.0835, -31.1004) (-117.0389, -31.0484) (-116.9947, -30.9963) (-116.9508, -30.9441) (-116.9072, -30.8917) (-116.8638, -30.8392) (-116.8208, -30.7865) (-116.7781, -30.7337) (-116.7357, -30.6808) (-116.6936, -30.6277) (-116.6518, -30.5745) (-116.6104, -30.5212) (-116.5692, -30.4677) (-116.5284, -30.414) (-116.4879, -30.3603) (-116.4478, -30.3063) (-116.408, -30.2523) (-116.3685, -30.1981) (-116.3293, -30.1438) (-116.2906, -30.0893) (-116.2521, -30.0347) (-116.214, -29.98) (-116.1763, -29.9251) (-116.1389, -29.8701) (-116.1019, -29.8149) (-116.0652, -29.7596) (-116.029, -29.7042) (-115.9931, -29.6486) (-115.9575, -29.5929) (-115.9224, -29.537) (-115.8877, -29.481) (-115.8534, -29.4249) (-115.8195, -29.3686) (-115.786, -29.3121) (-115.7529, -29.2556) (-115.7202, -29.1989) (-115.688, -29.142) (-115.6561, -29.085) (-115.6248, -29.0279) (-115.5939, -28.9706) (-115.5636, -28.9131) (-115.5337, -28.8555) (-115.5044, -28.7977) (-115.4755, -28.7398) (-115.4471, -28.6818) (-115.4191, -28.6236) (-115.3917, -28.5653) (-115.3647, -28.5068) (-115.3385, -28.4481) (-115.313, -28.3892) (-115.2883, -28.3301) (-115.2645, -28.2708) (-115.2414, -28.2113) (-115.2188, -28.1516) (-115.1967, -28.0919) (-115.1749, -28.0321) (-115.1537, -27.9721) (-115.1336, -27.9119) (-115.1152, -27.8513) (-115.1025, -27.8023) (-115.0942, -27.7653) (-115.0893, -27.7405) (-115.0871, -27.728) knots -1 -1 -1 -1 -1 -1 -0.98571429 -0.97142857 -0.95714286 -0.94285714 -0.92857143 -0.91428571 -0.9 -0.88571429 -0.87142857 -0.85714286 -0.84285714 -0.82857143 -0.81428571 -0.8 -0.78571429 -0.77142857 -0.75714286 -0.74285714 -0.72857143 -0.71428571 -0.7 -0.68571429 -0.67142857 -0.65714286 -0.64285714 -0.62857143 -0.61428571 -0.6 -0.58571429 -0.57142857 -0.55714286 -0.54285714 -0.52857143 -0.51428571 -0.5 -0.48571429 -0.47142857 -0.45714286 -0.44285714 -0.42857143 -0.41428571 -0.4 -0.38571429 -0.37142857 -0.35714286 -0.34285714 -0.32857143 -0.31428571 -0.3 -0.28571429 -0.27142857 -0.25714286 -0.24285714 -0.22857143 -0.21428571 -0.2 -0.18571429 -0.17142857 -0.15714286 -0.14285714 -0.12857143 -0.11428571 -0.1 -0.08571429 -0.07142857 -0.05714286 -0.04285714 -0.02857143 -0.01428571 0 0 0 0 0 0
  line L11 (-115.0871, -27.728) -> (-115.0688, -27.6286)
  arc A23 (-113.9399, -26.8197) -> (-115.0688, -27.6286) centre (-114.0852, -27.809) ccw
  arc A24 (-113.9399, -26.8197) -> (-113.1358, -26.9255) centre (-110, 0) ccw
  arc A25 (-112.2547, -27.9991) -> (-113.1358, -26.9255) centre (-113.2515, -27.9188) ccw
  line L12 (-112.2547, -27.9991) -> (-112.2628, -28.0998)
  spline S12 degree 5 poles (-112.2628, -28.0998) (-112.2638, -28.1124) (-112.2655, -28.1377) (-112.2672, -28.1756) (-112.2675, -28.2262) (-112.2655, -28.2895) (-112.2616, -28.3528) (-112.2567, -28.4162) (-112.2511, -28.4797) (-112.2452, -28.5431) (-112.2388, -28.6066) (-112.2319, -28.67) (-112.2242, -28.7335) (-112.2157, -28.797) (-112.2063, -28.8605) (-112.1962, -28.9239) (-112.1853, -28.9874) (-112.1738, -29.0508) (-112.1619, -29.1143) (-112.1495, -29.1777) (-112.1366, -29.2411) (-112.1232, -29.3045) (-112.1093, -29.3679) (-112.0948, -29.4312) (-112.0798, -29.4946) (-112.0643, -29.5579) (-112.0484, -29.6212) (-112.0319, -29.6844) (-112.015, -29.7477) (-111.9977, -29.8109) (-111.98, -29.8741) (-111.9618, -29.9372) (-111.9432, -30.0003) (-111.9241, -30.0634) (-111.9047, -30.1264) (-111.8848, -30.1895) (-111.8645, -30.2524) (-111.8438, -30.3154) (-111.8227, -30.3783) (-111.8012, -30.4411) (-111.7794, -30.504) (-111.7571, -30.5667) (-111.7345, -30.6295) (-111.7115, -30.6922) (-111.6881, -30.7548) (-111.6644, -30.8174) (-111.6402, -30.88) (-111.6158, -30.9425) (-111.5909, -31.005) (-111.5658, -31.0674) (-111.5402, -31.1297) (-111.5143, -31.1921) (-111.4881, -31.2543) (-111.4615, -31.3165) (-111.4346, -31.3787) (-111.4073, -31.4408) (-111.3797, -31.5029) (-111.3518, -31.5649) (-111.3236, -31.6268) (-111.295, -31.6887) (-111.2661, -31.7505) (-111.2368, -31.8123) (-111.2073, -31.874) (-111.1774, -31.9356) (-111.1472, -31.9972) (-111.1167, -32.0588) (-111.0858, -32.1202) (-111.0547, -32.1816) (-111.0233, -32.243) (-110.9915, -32.3043) (-110.9594, -32.3655) (-110.9336, -32.4144) (-110.914, -32.4511) (-110.9009, -32.4755) (-110.8943, -32.4877) knots 0 0 0 0 0 0 0.01428571 0.02857143 0.04285714 0.05714286 0.07142857 0.08571429 0.1 0.11428571 0.12857143 0.14285714 0.15714286 0.17142857 0.18571429 0.2 0.21428571 0.22857143 0.24285714 0.25714286 0.27142857 0.28571429 0.3 0.31428571 0.32857143 0.34285714 0.35714286 0.37142857 0.38571429 0.4 0.41428571 0.42857143 0.44285714 0.45714286 0.47142857 0.48571429 0.5 0.51428571 0.52857143 0.54285714 0.55714286 0.57142857 0.58571429 0.6 0.61428571 0.62857143 0.64285714 0.65714286 0.67142857 0.68571429 0.7 0.71428571 0.72857143 0.74285714 0.75714286 0.77142857 0.78571429 0.8 0.81428571 0.82857143 0.84285714 0.85714286 0.87142857 0.88571429 0.9 0.91428571 0.92857143 0.94285714 0.95714286 0.97142857 0.98571429 1 1 1 1 1 1
  arc A26 (-110.8943, -32.4877) -> (-109.1057, -32.4877) centre (-110, 0) ccw
  spline S13 degree 5 poles (-109.1057, -32.4877) (-109.0991, -32.4755) (-109.086, -32.4511) (-109.0664, -32.4144) (-109.0406, -32.3655) (-109.0085, -32.3043) (-108.9767, -32.243) (-108.9453, -32.1816) (-108.9142, -32.1202) (-108.8833, -32.0588) (-108.8528, -31.9972) (-108.8226, -31.9356) (-108.7927, -31.874) (-108.7632, -31.8123) (-108.7339, -31.7505) (-108.705, -31.6887) (-108.6764, -31.6268) (-108.6482, -31.5649) (-108.6203, -31.5029) (-108.5927, -31.4408) (-108.5654, -31.3787) (-108.5385, -31.3165) (-108.5119, -31.2543) (-108.4857, -31.1921) (-108.4598, -31.1297) (-108.4342, -31.0674) (-108.4091, -31.005) (-108.3842, -30.9425) (-108.3598, -30.88) (-108.3356, -30.8174) (-108.3119, -30.7548) (-108.2885, -30.6922) (-108.2655, -30.6295) (-108.2429, -30.5667) (-108.2206, -30.504) (-108.1988, -30.4411) (-108.1773, -30.3783) (-108.1562, -30.3154) (-108.1355, -30.2524) (-108.1152, -30.1895) (-108.0953, -30.1264) (-108.0759, -30.0634) (-108.0568, -30.0003) (-108.0382, -29.9372) (-108.02, -29.8741) (-108.0023, -29.8109) (-107.985, -29.7477) (-107.9681, -29.6844) (-107.9516, -29.6212) (-107.9357, -29.5579) (-107.9202, -29.4946) (-107.9052, -29.4312) (-107.8907, -29.3679) (-107.8768, -29.3045) (-107.8634, -29.2411) (-107.8505, -29.1777) (-107.8381, -29.1143) (-107.8262, -29.0508) (-107.8147, -28.9874) (-107.8038, -28.9239) (-107.7937, -28.8605) (-107.7843, -28.797) (-107.7758, -28.7335) (-107.7681, -28.67) (-107.7612, -28.6066) (-107.7548, -28.5431) (-107.7489, -28.4797) (-107.7433, -28.4162) (-107.7384, -28.3528) (-107.7345, -28.2895) (-107.7325, -28.2262) (-107.7328, -28.1756) (-107.7345, -28.1377) (-107.7362, -28.1124) (-107.7372, -28.0998) knots -1 -1 -1 -1 -1 -1 -0.98571429 -0.97142857 -0.95714286 -0.94285714 -0.92857143 -0.91428571 -0.9 -0.88571429 -0.87142857 -0.85714286 -0.84285714 -0.82857143 -0.81428571 -0.8 -0.78571429 -0.77142857 -0.75714286 -0.74285714 -0.72857143 -0.71428571 -0.7 -0.68571429 -0.67142857 -0.65714286 -0.64285714 -0.62857143 -0.61428571 -0.6 -0.58571429 -0.57142857 -0.55714286 -0.54285714 -0.52857143 -0.51428571 -0.5 -0.48571429 -0.47142857 -0.45714286 -0.44285714 -0.42857143 -0.41428571 -0.4 -0.38571429 -0.37142857 -0.35714286 -0.34285714 -0.32857143 -0.31428571 -0.3 -0.28571429 -0.27142857 -0.25714286 -0.24285714 -0.22857143 -0.21428571 -0.2 -0.18571429 -0.17142857 -0.15714286 -0.14285714 -0.12857143 -0.11428571 -0.1 -0.08571429 -0.07142857 -0.05714286 -0.04285714 -0.02857143 -0.01428571 0 0 0 0 0 0
  line L13 (-107.7372, -28.0998) -> (-107.7453, -27.9991)
  arc A27 (-106.8642, -26.9255) -> (-107.7453, -27.9991) centre (-106.7485, -27.9188) ccw
  arc A28 (-106.8642, -26.9255) -> (-106.0601, -26.8197) centre (-110, 0) ccw
  arc A29 (-104.9312, -27.6286) -> (-106.0601, -26.8197) centre (-105.9148, -27.809) ccw
  line L14 (-104.9312, -27.6286) -> (-104.9129, -27.728)